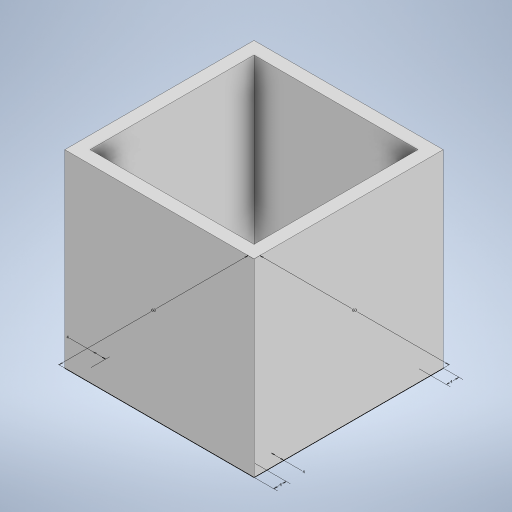
# Autodesk Inventor part: sensor_block
Saved by Autodesk Inventor 2024 (Build 280153000, 153)
## iProperties
Created: 2024-05-08
Part Number: sensor_block
Material: Generic
Document SubType Name: Modeling
Designer: kamil
Density: 1 g/cm^3
Appearance: Default
Author: kamil
Autodesk Inventor part; units mm, degrees
ref_plane "YZ Plane" through (0, 0, 0) normal (1, 0, 0) x (0, 1, 0)
ref_plane "XZ Plane" through (0, 0, 0) normal (0, 1, 0) x (-1, 0, 0)
ref_plane "XY Plane" through (0, 0, 0) normal (0, 0, 1) x (1, 0, 0)
sketch "Sketch1" plane through (0, 0, 0) normal (0, 1, 0) x (-1, 0, 0)
  line L0 (0, 0) -> (60, 0)
  line L1 (60, 0) -> (60, -60)
  line L2 (60, -60) -> (0, -60)
  line L3 (0, -60) -> (0, 0)
  line L4 (4, -4) -> (56, -4)
  line L5 (56, -4) -> (56, -56)
  line L6 (56, -56) -> (4, -56)
  line L7 (4, -56) -> (4, -4)
  dimension "d0" = 60
  dimension "d1" = 60
  dimension "d2" = 4
  dimension "d3" = 4
  dimension "d4" = 4
  dimension "d5" = 4
  constraints: 16 end point, 4 parallel, 2 horizontal, 2 perpendicular
  measures "d0" distance of L1.end L2.end
  measures "d1" distance of L0.end L1.end
  measures "d2" distance between parallel lines of L4 L0
  measures "d3" distance between parallel lines of L3 L7
  measures "d4" distance between parallel lines of L1 L5
  measures "d5" distance between parallel lines of L2 L6
extrude "Extrusion1" add sketch "Sketch1" along normal blind 4 contours L4 L5 L6 L7
extrude "Extrusion2" add sketch "Sketch1" along normal blind 60
body "Solid1"
